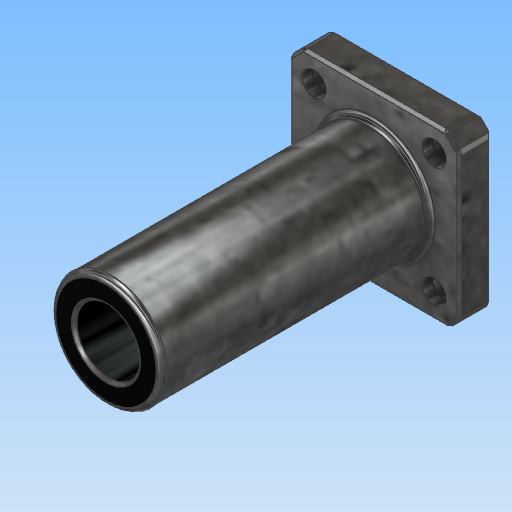
# Autodesk Inventor part: LMK16LUU
Saved by Autodesk Inventor 2017 (Build 210142000, 142)
## iProperties
Part Number: LMK16LUU
Material: Типовые
Document SubType Name: Modeling
Designer: alcapone
Density: 1 g/cm^3
Appearance: Сталь - гальванизированная
Mass: 16.1955 g
Surface Area: 81.9505 cm^2
Volume: 16.1955 cm^3
Author: alcapone
Autodesk Inventor part; units mm, degrees
ref_plane "YZ Plane" through (0, 0, 0) normal (1, 0, 0) x (0, 1, 0)
ref_plane "XZ Plane" through (0, 0, 0) normal (0, 1, 0) x (-1, 0, 0)
ref_plane "XY Plane" through (0, 0, 0) normal (0, 0, 1) x (1, 0, 0)
sketch "Эскиз1" plane through (0, 0, 0) normal (0, 0, 1) x (1, 0, 0)
  circle A0 centre (0, 0) radius 6
  circle A1 centre (0, 0) radius 10.5
  circle A2 centre (0, 0) radius 16 construction
  line L0 (13.8701, -16) -> (-13.8701, -16)
  line L1 (-16, -13.8701) -> (-16, 13.5269)
  line L2 (-13.5269, 16) -> (13.5269, 16)
  line L3 (16, 13.5269) -> (16, -13.8701)
  line L4 (20.7678, -20.7678) -> (-17.2322, 17.2322) construction
  line L5 (-19, -19) -> (19, 19) construction
  line L6 (-16, 13.5269) -> (-13.5269, 16)
  line L7 (13.5269, 16) -> (16, 13.5269)
  line L8 (16, -13.8701) -> (13.8701, -16)
  line L9 (-13.8701, -16) -> (-16, -13.8701)
  line L10 (0, 0) -> (60, 0) construction
  line L11 (0, 0) -> (0, 33.9896) construction
  circle A3 centre (-11.3137, 11.3137) radius 2.25
  circle A4 centre (-11.3137, 11.3137) radius 3.75
  circle A5 centre (-11.3137, -11.3137) radius 2.25
  circle A6 centre (-11.3137, -11.3137) radius 3.75
  circle A7 centre (11.3137, -11.3137) radius 2.25
  circle A8 centre (11.3137, -11.3137) radius 3.75
  circle A9 centre (11.3137, 11.3137) radius 2.25
  circle A10 centre (11.3137, 11.3137) radius 3.75
  circle A11 centre (0, 0) radius 9.5
  dimension "d2" = 32
  dimension "d0" = 12
  dimension "d1" = 21
  dimension "d3" = 32
  dimension "d14" = 4.5
  dimension "d15" = 7.5
  dimension "d18" = 360
  dimension "d24" = 19
  dimension "d38" = 32
  dimension "d39" = 42
  dimension "d40" = 42
  constraints: 24 end point, 11 centre point, 8 coincident, 4 perpendicular, 2 horizontal, 2 parallel, 2 point on line, 1 midpoint, 1 vertical, 24 other
  measures "d0" diameter of A0
  measures "d1" diameter of A1
  measures "d3" distance between parallel lines of L3 L1
  measures "d14" diameter of A3
  measures "d15" diameter of A4
  measures "d24" diameter of A11
  measures "d38" distance between parallel lines of L0 L2
  measures "d39" distance between parallel lines of L8 L6
  measures "d40" distance between parallel lines of L7 L9
extrude "Выдавливание1" add sketch "Эскиз1" along normal blind 57 contours A1 | A11
extrude "Выдавливание2" add sketch "Эскиз1" along normal blind 6 contours L0 L9 L1 L6 L2 L7 L3 L8 | A3 | A4 | A5 | A6 | A7 | A8 | A9 | A10
extrude "Выдавливание3" cut sketch "Эскиз1" along normal blind 6 contours A3 | A5 | A7 | A9
extrude "Выдавливание4" cut sketch "Эскиз1" along normal blind 4.1 contours A4 | A6 | A8 | A10
extrude "Выдавливание5" cut sketch "Эскиз1" along normal blind 0.5 contours A11
sketch "Эскиз2" plane through (0, 0, 57) normal (0, 0, 1) x (1, 0, 0)
  circle A0 centre (0, 0) radius 13
  dimension "d27" = 26
  constraints: 1 centre point, 1 coincident
  measures "d27" diameter of A0
extrude "Выдавливание6" cut sketch "Эскиз2" against normal blind 0.5
chamfer "Фаска1" distance 0.5 angle 45 2 edges at (-6, 0, 56.5) (-6, 0, 0.5)
fillet "Сопряжение2" radius 1 1 edges at (-10.5, 0, 6)
chamfer "Фаска2" distance 0.5 angle 45 27 edges at (-16, -0.1716, 6) (-14.935, -14.935, 6) (0, -16, 6) (0, 16, 6) (-14.7635, 14.7635, 6) (16, -0.1716, 6) (14.7635, 14.7635, 6) (-16, 13.5269, 3) (-13.5269, 16, 3) (16, 13.5269, 3) (13.5269, 16, 3) (0, 16, 0) (-14.7635, 14.7635, 0) (16, -0.1716, 0) (14.935, -14.935, 6) (13.8701, -16, 3) (-13.8701, -16, 3) (0, -16, 0) (14.935, -14.935, 0) (16, -13.8701, 3) (-14.935, -14.935, 0) (-16, -13.8701, 3) (-16, -0.1716, 0) (-15.0637, -11.3137, 0) (-15.0637, 11.3137, 0) (7.5637, 11.3137, 0) (7.5637, -11.3137, 0)
fillet "Сопряжение3" radius 1 1 edges at (-10.5, 0, 56.5)
